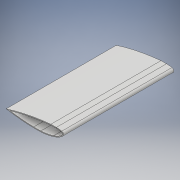
# Autodesk Inventor part: GFRP_mc
Saved by Autodesk Inventor 2018.2 (Build 222227000, 227)
## iProperties
Created: 2018-04-22
Part Number: GFRP_mc
Material: 一般
Document SubType Name: Modeling
Designer: ku_sk
Density: 1 g/cm^3
Appearance: 既定
Author: ku_sk
Autodesk Inventor part; units mm, degrees
ref_plane "YZ Plane" through (0, 0, 0) normal (1, 0, 0) x (0, 1, 0)
ref_plane "XZ Plane" through (0, 0, 0) normal (0, 1, 0) x (-1, 0, 0)
ref_plane "XY Plane" through (0, 0, 0) normal (0, 0, 1) x (1, 0, 0)
sketch "スケッチ1" plane through (0, 0, 0) normal (0, 1, 0) x (-1, 0, 0)
  arc A0 (99.4141, -32.927) -> (197.8245, -22.9934) centre (88.5018, 567.6156) ccw projected
  arc A1 (73.8469, -32.6347) -> (99.4141, -32.927) centre (91.566, 398.982) ccw projected
  arc A2 (27.3573, -24.3709) -> (73.8469, -32.6347) centre (81.048, 142.776) ccw projected
  arc A3 (0.844, -11.3484) -> (27.3573, -24.3709) centre (58.458, 72.45) ccw projected
  arc A4 (-6.1834, -4.5246) -> (0.844, -11.3484) centre (17.4, 12.732) ccw projected
  arc A5 (-1.3535, 7.5415) -> (-6.1834, -4.5246) centre (0, 0) ccw projected
  arc A6 (18.2937, 9.3227) -> (-1.3535, 7.5415) centre (18.66, -103.968) ccw projected
  arc A7 (38.1205, 9.1058) -> (18.2937, 9.3227) centre (20.556, -690.396) ccw projected
  arc A8 (197.8245, -22.9934) -> (38.1205, 9.1058) centre (-36.3979, -774.9853) ccw projected
  circle A9 centre (20, -2.2582) radius 6 projected
  circle A10 centre (130, -14.678) radius 6 projected
extrude "押し出し1" add sketch "スケッチ1" along normal mid plane 394 contours A1 A2 A3 A4 A5 A6 A7 A8 A0 | A9 | A10
shell "シェル1" thickness 3 removed faces 2 at (-50.4147, -197, -4.6886) at (-50.4147, 197, -4.6886)
